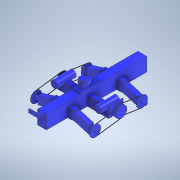
# Autodesk Inventor part: chassis
Saved by Autodesk Inventor 2021 (Build 250183000, 183)
## iProperties
Created: 2020-11-19
Part Number: chassis
Material: Generic
Document SubType Name: Modeling
Designer: Mateusz
Density: 1 g/cm^3
Appearance: Default
Author: Mateusz
Autodesk Inventor part; units mm, degrees
ref_plane "YZ Plane" through (0, 0, 0) normal (1, 0, 0) x (0, 1, 0)
ref_plane "XZ Plane" through (0, 0, 0) normal (0, 1, 0) x (-1, 0, 0)
ref_plane "Work Plane1" through (-479.9998, 3, -645.0001) normal (0, 1, 0) x (1, 0, 0)
sketch "Sketch1" plane through (-479.9998, 3, -645.0001) normal (0, 1, 0) x (1, 0, 0)
  line L0 (-140.0002, -474.9989) -> (-260.0002, -474.9989)
  line L1 (-260.0002, -474.9989) -> (-260.0002, -514.9996)
  line L2 (-260.0002, -514.9996) -> (-380.0002, -544.9996)
  line L3 (-380.0002, -544.9996) -> (-380.0002, -625.0004)
  line L4 (-380.0002, -625.0004) -> (240.0001, -625.0004)
  line L5 (240.0001, -625.0004) -> (240.0001, -545.0003)
  line L6 (240.0001, -545.0003) -> (120.0001, -515.0003)
  line L7 (120.0001, -515.0003) -> (120.0001, -474.9989)
  line L8 (120.0001, -474.9989) -> (0, -474.9989)
  line L9 (0, -474.9989) -> (0.0003, -419.9989)
  line L10 (0.0003, -419.9989) -> (0.0003, -349.9996)
  line L11 (0.0003, -349.9996) -> (-0.0003, -295.0009)
  line L12 (-0.0003, -295.0009) -> (120.0001, -294.9996)
  line L13 (120.0001, -294.9996) -> (120.0001, -255.0003)
  line L14 (120.0001, -255.0003) -> (240, -225)
  line L15 (240, -225) -> (240, -125)
  line L16 (240, -125) -> (120, -95)
  line L17 (120, -95) -> (120, 0)
  line L18 (120, 0) -> (0, 0)
  line L19 (0, 0) -> (0, 70)
  line L20 (0, 70) -> (120, 70)
  line L21 (120, 70) -> (120, 165)
  line L22 (120, 165) -> (240, 195)
  line L23 (240, 195) -> (240, 274.9997)
  line L24 (240, 274.9997) -> (-380.0002, 274.9997)
  line L25 (-380.0002, 274.9997) -> (-380.0002, 194.9997)
  line L26 (-380.0002, 194.9997) -> (-260.0002, 164.9996)
  line L27 (-260.0002, 164.9996) -> (-260.0002, 99.9996)
  line L28 (-260.0002, 99.9996) -> (-260.0002, 70)
  line L29 (-260.0002, 70) -> (-140.0002, 70)
  line L30 (-140.0002, 70) -> (-140.0002, 0)
  line L31 (-140.0002, 0) -> (-260.0002, 0)
  line L32 (-260.0002, 0) -> (-260.0002, -30)
  line L33 (-260.0002, -30) -> (-260.0002, -94.9996)
  line L34 (-260.0002, -94.9996) -> (-380.0002, -124.9996)
  line L35 (-380.0002, -124.9996) -> (-380.0002, -224.9996)
  line L36 (-380.0002, -224.9996) -> (-260.0002, -254.9996)
  line L37 (-260.0002, -254.9996) -> (-260.0002, -294.9996)
  line L38 (-260.0002, -294.9996) -> (-140.0002, -294.9996)
  line L39 (-140.0002, -294.9996) -> (-140.0002, -474.9989)
extrude "Extrusion1" add sketch "Sketch1" along normal blind 3
sketch "Sketch2" plane through (-479.9998, 6, -645.0001) normal (0, 1, 0) x (1, 0, 0)
  line L0 (240, 274.9997) -> (-380.0002, 274.9997) projected
  line L1 (-70.0001, -588.0003) -> (-107.7001, -588.0003)
  line L2 (-107.7001, -588.0003) -> (-32.3001, -588.0003)
  line L3 (-32.3001, -588.0003) -> (-32.3001, 274.9997)
  line L4 (-107.7001, -588.0003) -> (-107.7001, 274.9997)
  line L5 (-32.3001, 274.9997) -> (-107.7001, 274.9997)
  point P0 (479.9998, -645.0001)
  dimension "d4" = 37.7
  dimension "d5" = 75.4
  constraints: 10 end point, 3 point on line, 2 perpendicular, 1 collinear, 1 horizontal
  measures "d4" distance of L1.start L1.end
  measures "d5" distance of L1.end L2.end
extrude "Extrusion2" add sketch "Sketch2" along normal blind 115.4
sketch "Sketch3" plane through (-479.9998, 6, -645.0001) normal (0, 1, 0) x (1, 0, 0)
  line L0 (-140.0002, -404.9993) -> (-107.7001, -404.9993)
  line L1 (-107.7001, -588.0003) -> (-107.7001, 274.9997) projected
  line L2 (-140.0002, -364.9993) -> (0.0003, -364.9993)
  line L3 (0.0003, -404.9993) -> (-107.7001, -404.9993)
  line L4 (0, 15) -> (-140.0002, 15)
  line L5 (-140.0002, 55) -> (0, 55)
  line L6 (-70, -364.9993) -> (28.5, -364.9993)
  line L7 (28.5, -364.9993) -> (-168.5, -364.9993)
  line L8 (-168.5, -364.9993) -> (-168.5, -404.9993)
  line L9 (-168.5, -404.9993) -> (-140.0002, -404.9993)
  line L10 (0.0003, -404.9993) -> (28.5, -404.9993)
  line L11 (28.5, -404.9993) -> (28.5, -364.9993)
  line L12 (0, 55) -> (28.5, 55)
  line L13 (28.5, 55) -> (28.5, 15)
  line L14 (28.5, 15) -> (0, 15)
  line L15 (0, 0) -> (0, 70) projected
  line L16 (-140.0002, 55) -> (-168.5, 55)
  line L17 (-168.5, 55) -> (-168.5, 15)
  line L18 (-168.5, 15) -> (-140.0002, 15)
  point P0 (479.9998, -645.0001)
  dimension "d12" = 40
  dimension "d19" = 98.5
  dimension "d20" = 197
  constraints: 34 end point, 7 point on line, 6 perpendicular, 1 collinear, 1 horizontal, 1 midpoint, 1 parallel
  measures "d12" distance of L4.end L5.start
  measures "d19" distance of L6.start L6.end
  measures "d20" distance of L6.end L7.end
extrude "Extrusion3" add sketch "Sketch3" along normal blind 78.5
sketch "Sketch4" plane through (-479.9998, 6, -645.0001) normal (0, 1, 0) x (1, 0, 0)
  line L0 (0.0003, -404.9993) -> (0.0003, -364.9993) projected
  line L1 (0.0003, -384.9993) -> (0.0003, -349.9993)
  line L2 (0.0003, -349.9993) -> (0.0003, -419.9993)
  line L3 (0, -474.9989) -> (0.0003, -419.9989) projected
  line L4 (0.0003, -419.9993) -> (120.0001, -419.9993)
  line L5 (120.0001, -474.9989) -> (0, -474.9989) projected
  line L6 (120.0001, -419.9993) -> (120.0001, -474.9989)
  line L7 (120.0001, -474.9989) -> (0, -474.9989)
  line L8 (0, -474.9989) -> (0.0003, -419.9993)
  line L9 (0.0003, -419.9989) -> (0.0003, -349.9996) projected
  line L10 (0.0003, -349.9996) -> (-0.0003, -295.0009) projected
  line L11 (0.0003, -349.9996) -> (-0.0003, -295.0009)
  line L12 (-0.0003, -295.0009) -> (120.0001, -294.9996) projected
  line L13 (-0.0003, -295.0009) -> (120.0001, -294.9996)
  line L14 (120.0001, -294.9996) -> (120.0001, -349.9996)
  line L15 (120.0001, -349.9996) -> (0.0003, -349.9996)
  line L16 (-140.0002, -364.9993) -> (-140.0002, -404.9993) projected
  line L17 (-140.0002, -384.9993) -> (-140.0002, -349.9996)
  line L18 (-140.0002, -294.9996) -> (-140.0002, -474.9989) projected
  line L19 (-140.0002, -384.9993) -> (-140.0002, -419.9993)
  line L20 (-140.0002, -294.9996) -> (-140.0002, -474.9989) projected
  arc A0 (-140.0002, -419.9993) -> (-140.0002, -419.9993) centre (-140.0002, 50751.7356) ccw
  line L21 (-140.0002, -419.9993) -> (-140.0002, -474.9989)
  line L22 (-140.0002, -474.9989) -> (-260.0002, -474.9989) projected
  line L23 (-260.0002, -474.9989) -> (-260.0002, -514.9996) projected
  line L24 (-140.0002, -474.9989) -> (-260.0002, -474.9989)
  line L25 (-260.0002, -474.9989) -> (-260.0002, -419.9993)
  line L26 (-260.0002, -419.9993) -> (-140.0002, -419.9993)
  line L27 (-140.0002, -349.9996) -> (-140.0002, -294.9996)
  line L28 (-260.0002, -294.9996) -> (-140.0002, -294.9996) projected
  line L29 (-140.0002, -294.9996) -> (-260.0002, -294.9996)
  line L30 (-260.0002, -294.9996) -> (-260.0002, -349.9996)
  line L31 (-260.0002, -349.9996) -> (-140.0002, -349.9996)
  point P0 (479.9998, -645.0001)
  dimension "d15" = 35
  dimension "d16" = 70
  constraints: 40 end point, 9 point on line, 7 perpendicular, 5 collinear, 2 midpoint, 2 point on circle, 1 centre point, 1 horizontal
  measures "d15" distance of L1.start L1.end
  measures "d16" distance of L1.end L2.end
extrude "Extrusion4" add sketch "Sketch4" against normal up to surface (3 mm away) contours L10 L12 L14 L15 | L31 L30 L28 L18 | L4 L6 L5 L3 | L18 L22 L25 L26
sketch "Sketch5" plane through (-479.9995, 6, -240.0008) normal (0, 0, 1) x (1, 0, 0)
  line L0 (0, 0) -> (28.4997, 0) projected
  line L1 (28.4997, 78.5) -> (-32.3004, 78.5) projected
  line L2 (28.4997, 78.5) -> (28.4997, 68.5)
  line L3 (28.4997, 0) -> (28.4997, 78.5) projected
  line L4 (28.4997, 68.5) -> (150.0967, 31.842)
  line L5 (28.4997, 0) -> (150.0967, -36.658)
  line L6 (150.0967, -36.658) -> (150.0967, 31.842)
  line L7 (28.4997, 68.5) -> (28.4997, 0)
  line L8 (-107.7004, 115.4) -> (-32.3004, 115.4) projected
  line L9 (-70.0004, 115.4) -> (-70.0004, 84.9385)
  line L10 (-140.0008, 0) -> (-168.5005, 0)
  line L11 (-168.5005, 78.5) -> (-107.7004, 78.5)
  line L12 (-168.5005, 78.5) -> (-168.5005, 68.5)
  line L13 (-168.5005, 0) -> (-168.5005, 78.5)
  line L14 (-168.5005, 68.5) -> (-290.0975, 31.842)
  line L15 (-168.5005, 0) -> (-290.0975, -36.658)
  line L16 (-290.0975, -36.658) -> (-290.0975, 31.842)
  line L17 (-168.5005, 68.5) -> (-168.5005, 0)
  point P0 (479.9995, -6)
  dimension "d24" = 10
  constraints: 28 end point, 7 symmetric about line, 2 point on line, 2 vertical, 1 collinear, 1 midpoint, 1 parallel
  measures "d24" distance of L1.start L2.end
extrude "Extrusion5" add sketch "Sketch5" against normal up to surface (40 mm away)
sketch "Sketch6" plane through (-479.9998, 6, -660.0001) normal (0, 0, 1) x (1, 0, 0)
  line L0 (-32.3001, 0) -> (-32.3001, 78.5) projected
  line L1 (0.0003, 0) -> (-32.3001, 0) projected
  line L2 (0.0003, 0) -> (28.5, 0) projected
  line L3 (28.5, 0) -> (150.097, -36.658) projected
  line L4 (150.097, -36.658) -> (150.097, 31.842) projected
  line L5 (150.097, 31.842) -> (28.5, 68.5) projected
  line L6 (28.5, 68.5) -> (28.5, 78.5) projected
  line L7 (-32.3001, 78.5) -> (28.5, 78.5) projected
  line L8 (-290.0972, -36.658) -> (-168.5002, 0) projected
  line L9 (-168.5002, 0) -> (-168.5002, 68.5) projected
  line L10 (-168.5002, 68.5) -> (-290.0972, 31.842) projected
  line L11 (-290.0972, 31.842) -> (-290.0972, -36.658) projected
  point P0 (479.9998, -6)
extrude "Extrusion6" add sketch "Sketch6" against normal up to surface (40 mm away)
sketch "Sketch8" plane through (-479.9998, 121.4, -645.0001) normal (0, 1, 0) x (1, 0, 0)
  line L0 (240, -225) -> (240, -125) projected
  line L1 (240, -175) -> (-32.3001, -174.9996)
  line L2 (-32.3001, 15) -> (-32.3001, -364.9993) projected
  line L3 (-32.3001, -174.9996) -> (-107.7001, -174.9996)
  line L4 (-107.7001, -364.9993) -> (-107.7001, 15) projected
  circle A0 centre (-70.0001, -174.9996) radius 14.9657
  line L5 (-70.0001, -174.9996) -> (-70.0001, -224.9996)
  circle A1 centre (-70.0001, -224.9996) radius 8.3807
  line L6 (-107.7001, 274.9997) -> (-107.7001, -588.0003) projected
  line L7 (-32.3001, -588.0003) -> (-32.3001, 274.9997) projected
  line L8 (-107.7001, -253.6114) -> (-32.3001, -253.6114)
  line L9 (-32.3001, -253.6114) -> (-32.3001, -135.5582)
  line L10 (-32.3001, -135.5582) -> (-107.7001, -135.5582)
  line L11 (-107.7001, -135.5582) -> (-107.7001, -253.6114)
  point P0 (479.9998, -645.0001)
  point P1 (-32.3001, -135.5582)
  point P2 (-107.7001, -135.5582)
  point P3 (-107.7001, -253.6114)
  point P4 (-32.3001, -253.6114)
  dimension "d30" = 50
  constraints: 14 end point, 4 midpoint, 2 centre point, 2 parallel, 2 point on line, 1 coincident, 1 horizontal, 1 perpendicular, 1 vertical
  measures "d30" distance of L5.start L5.end
extrude "Extrusion7" add sketch "Sketch8" along normal blind 13.941 contours L2 L3 A0 L4 L10 | A1 | L2 L8 L4 L3 A0 | A0 L5 L3 | L3 A0 | L5 A0 L3
sketch "Sketch9" plane through (-587.6999, 6, -56.9998) normal (0, 0, 1) x (1, 0, 0)
  line L0 (0, 115.4) -> (75.4, 115.4) projected
  line L1 (37.7, 85.538) -> (47.7, 85.538)
  line L2 (47.7, 85.538) -> (37.7, 85.538)
  line L3 (37.7, 85.538) -> (27.7, 85.538)
  line L4 (27.7, 85.538) -> (27.7, 115.4)
  line L5 (47.7, 85.538) -> (47.7, 115.4)
  line L6 (47.7, 115.4) -> (27.7, 115.4)
  point P0 (587.6999, -6)
  constraints: 12 end point, 3 perpendicular, 3 point on line, 1 collinear, 1 horizontal
extrude "Extrusion8" add sketch "Sketch9" along normal blind 30
sketch "Sketch10" plane through (-587.6999, 6, -26.9998) normal (0, 0, 1) x (1, 0, 0)
  line L0 (47.7, 115.4) -> (27.7, 115.4) projected
  line L1 (47.7, 115.4) -> (53.2, 115.4)
  line L2 (47.7, 115.4) -> (75.4, 115.4) projected
  line L3 (53.2, 115.4) -> (53.2, 85.538)
  line L4 (53.2, 85.538) -> (-40.3, 85.538)
  line L5 (-40.3, 85.538) -> (-40.3, 115.4)
  line L6 (-40.3, 115.4) -> (47.7, 115.4)
  point P0 (587.6999, -6)
  dimension "d39" = 5.5
  dimension "d40" = 93.5
  constraints: 10 end point, 2 perpendicular, 1 collinear, 1 horizontal, 1 point on line
  measures "d39" distance of L0.start L1.end
  measures "d40" distance of L3.end L4.end
extrude "Extrusion9" add sketch "Sketch10" along normal blind 7
sketch "Sketch11" plane through (-479.9998, 6, -645.0001) normal (0, 1, 0) x (1, 0, 0)
  line L0 (-107.7001, -404.9993) -> (-140.0002, -404.9993) projected
  line L1 (-140.0002, -404.9993) -> (-140.0002, -419.9993) projected
  line L2 (-140.0002, -419.9993) -> (-260.0002, -419.9993) projected
  line L3 (-260.0002, -419.9993) -> (-260.0002, -514.9996) projected
  line L4 (-260.0002, -514.9996) -> (-380.0002, -544.9996) projected
  line L5 (-380.0002, -544.9996) -> (-380.0002, -625.0004) projected
  line L6 (-380.0002, -625.0004) -> (240.0001, -625.0004) projected
  line L7 (240.0001, -625.0004) -> (240.0001, -545.0003) projected
  line L8 (240.0001, -545.0003) -> (120.0001, -515.0003) projected
  line L9 (120.0001, -515.0003) -> (120.0001, -419.9993) projected
  line L10 (120.0001, -419.9993) -> (0.0003, -419.9993) projected
  line L11 (0.0003, -419.9993) -> (0.0003, -419.9989) projected
  line L12 (0.0003, -419.9989) -> (0.0003, -404.9993) projected
  line L13 (0.0003, -404.9993) -> (-32.3001, -404.9993) projected
  line L14 (-32.3001, -404.9993) -> (-32.3001, -588.0003) projected
  line L15 (-32.3001, -588.0003) -> (-107.7001, -588.0003) projected
  line L16 (-107.7001, -588.0003) -> (-107.7001, -404.9993) projected
  line L17 (-107.7001, 15) -> (-140.0002, 15) projected
  line L18 (-140.0002, 15) -> (-140.0002, 0) projected
  line L19 (-140.0002, 0) -> (-260.0002, 0) projected
  line L20 (-260.0002, 0) -> (-260.0002, -94.9996) projected
  line L21 (-260.0002, -94.9996) -> (-380.0002, -124.9996) projected
  line L22 (-380.0002, -124.9996) -> (-380.0002, -224.9996) projected
  line L23 (-380.0002, -224.9996) -> (-260.0002, -254.9996) projected
  line L24 (-260.0002, -254.9996) -> (-260.0002, -349.9996) projected
  line L25 (-260.0002, -349.9996) -> (-140.0002, -349.9996) projected
  line L26 (-140.0002, -349.9996) -> (-140.0002, -364.9993) projected
  line L27 (-140.0002, -364.9993) -> (-107.7001, -364.9993) projected
  line L28 (-107.7001, -364.9993) -> (-107.7001, 15) projected
  line L29 (-140.0002, 55) -> (-107.7001, 55) projected
  line L30 (-107.7001, 55) -> (-107.7001, 274.9997) projected
  line L31 (-107.7001, 274.9997) -> (-380.0002, 274.9997) projected
  line L32 (-380.0002, 274.9997) -> (-380.0002, 194.9997) projected
  line L33 (-380.0002, 194.9997) -> (-260.0002, 164.9996) projected
  line L34 (-260.0002, 164.9996) -> (-260.0002, 70) projected
  line L35 (-260.0002, 70) -> (-140.0002, 70) projected
  line L36 (-140.0002, 70) -> (-140.0002, 55) projected
  line L37 (-32.3001, 55) -> (0, 55) projected
  line L38 (0, 55) -> (0, 70) projected
  line L39 (0, 70) -> (120, 70) projected
  line L40 (120, 70) -> (120, 165) projected
  line L41 (120, 165) -> (240, 195) projected
  line L42 (240, 195) -> (240, 274.9997) projected
  line L43 (240, 274.9997) -> (-32.3001, 274.9997) projected
  line L44 (-32.3001, 274.9997) -> (-32.3001, 55) projected
  line L45 (0, 15) -> (-32.3001, 15) projected
  line L46 (-32.3001, 15) -> (-32.3001, -364.9993) projected
  line L47 (-32.3001, -364.9993) -> (0.0003, -364.9993) projected
  line L48 (0.0003, -364.9993) -> (0.0003, -349.9996) projected
  line L49 (0.0003, -349.9996) -> (120.0001, -349.9996) projected
  line L50 (120.0001, -349.9996) -> (120.0001, -255.0003) projected
  line L51 (120.0001, -255.0003) -> (240, -225) projected
  line L52 (240, -225) -> (240, -125) projected
  line L53 (240, -125) -> (120, -95) projected
  line L54 (120, -95) -> (120, 0) projected
  line L55 (120, 0) -> (0, 0) projected
  line L56 (0, 0) -> (0, 15) projected
  point P0 (479.9998, -645.0001)
extrude "Extrusion10" cut sketch "Sketch11" against normal up to surface (3 mm away)
sketch "Sketch13" plane through (-479.9998, 121.4, -645.0001) normal (0, 1, 0) x (1, 0, 0)
  line L0 (-32.3001, -253.6114) -> (-107.7001, -253.6114) projected
  line L1 (-32.3001, -253.6114) -> (-32.3001, -293.6114)
  line L2 (-32.3001, -588.0003) -> (-32.3001, -253.6114) projected
  line L3 (-32.3001, -293.6114) -> (-107.7001, -293.6114)
  line L4 (-107.7001, -364.9993) -> (-107.7001, 15) projected
  line L5 (-107.7001, -253.6114) -> (-107.7001, -293.6114)
  point P0 (479.9998, -645.0001)
  dimension "d45" = 40
  constraints: 6 end point, 3 point on line, 1 collinear, 1 perpendicular
  measures "d45" distance of L0.start L1.end
extrude "Extrusion11" add sketch "Sketch13" along normal up to surface (13.941 mm away)
sketch "Sketch14" plane through (-479.9998, 135.341, -645.0001) normal (0, 1, 0) x (1, 0, 0)
  line L0 (-32.3001, -293.6114) -> (-107.7001, -293.6114) projected
  circle A0 centre (-70.0001, -237.6499) radius 30.3987
  circle A1 centre (-70.0001, -178.6114) radius 12.4726
  line L1 (-98.9637, -228.4198) -> (-81.8838, -174.8243)
  line L2 (-41.0365, -228.4198) -> (-58.1164, -174.8243)
  point P0 (479.9998, -645.0001)
  constraints: 4 end point, 4 point on circle, 4 tangent, 2 centre point, 1 other
extrude "Extrusion12" add sketch "Sketch14" along normal blind 40
sketch "Sketch15" plane through (-479.9998, 175.341, -645.0001) normal (0, 1, 0) x (1, 0, 0)
  arc A0 (-98.9637, -228.4198) -> (-41.0365, -228.4198) centre (-70.0001, -237.6499) ccw projected
  circle A1 centre (-70.0001, -237.6499) radius 27.858
  point P0 (479.9998, -645.0001)
  constraints: 1 centre point, 1 coincident
extrude "Extrusion13" add sketch "Sketch15" along normal blind 20
sketch "Sketch16" plane through (-587.6999, 3, -56.9998) normal (-1, 0, 0) x (0, 0, 1)
  line L0 (-223.0011, 3) -> (-223.0011, 81.5) projected
  line L1 (-223.0011, 81.5) -> (-353.0011, 81.5)
  line L2 (-353.0011, 81.5) -> (-353.0011, 0)
  line L3 (-603.0003, 0) -> (-223.0011, 0) projected
  line L4 (-353.0011, 81.5) -> (-393.0011, 81.5)
  line L5 (-393.0011, 81.5) -> (-393.0011, 0)
  line L6 (-353.0011, 0) -> (-393.0011, 0)
  point P0 (56.9998, -3)
  dimension "d55" = 130
  dimension "d56" = 40
  constraints: 10 end point, 3 perpendicular, 3 point on line, 1 horizontal
  measures "d55" distance of L0.end L1.end
  measures "d56" distance of L1.end L4.end
extrude "Extrusion14" add sketch "Sketch16" along normal up to surface (182.3971 mm away)
sketch "Sketch17" plane through (-770.097, 3, -450.0008) normal (-1, 0, 0) x (0, 0, 1)
  line L0 (40, 0) -> (0, 0) projected
  line L1 (40, 0) -> (40, 90)
  line L2 (40, 90) -> (-85, 90)
  line L3 (-85, 90) -> (-85, 0)
  line L4 (-209.9993, 0) -> (170, 0) projected
  line L5 (40, 0) -> (-85, 0)
  point P0 (450.0008, -3)
  dimension "d59" = 90
  dimension "d60" = 125
  constraints: 8 end point, 3 perpendicular, 1 point on line, 1 vertical
  measures "d59" distance of L0.start L1.end
  measures "d60" distance of L1.end L2.end
extrude "Extrusion15" add sketch "Sketch17" against normal blind 3
sketch "Sketch18" plane through (-587.6999, 3, -410.0008) normal (0, 0, 1) x (1, 0, 0)
  line L0 (-179.3971, 0) -> (-179.3971, 81.5) projected
  line L1 (0, 81.5) -> (-179.3971, 81.5) projected
  line L2 (-179.3971, 81.5) -> (-149.3971, 81.5)
  circle A0 centre (-149.3971, 81.5) radius 30
  point P0 (587.6999, -3)
  dimension "d64" = 30
  constraints: 2 end point, 1 coincident, 1 horizontal alignment, 1 point on line, 2 other
  measures "d64" distance of L0.end L2.end
extrude "Extrusion16" add sketch "Sketch18" along normal blind 60
extrude "Extrusion17" add sketch "Sketch18" against normal blind 100
sketch "Sketch19" plane through (-512.2999, 3, -919.9998) normal (1, 0, 0) x (0, 0, -1)
  line L0 (-469.9989, 81.5) -> (-509.9989, 81.5) projected
  line L1 (-469.9989, 0) -> (-469.9989, 81.5) projected
  line L2 (-509.9989, 81.5) -> (-509.9989, 0) projected
  line L3 (-469.9989, 0) -> (-259.9997, 0) projected
  line L4 (-219.9997, 0) -> (-259.9997, 0) projected
  line L5 (-219.9997, 0) -> (0, 0) projected
  line L6 (0, 0) -> (-219.9997, 0) projected
  line L7 (-259.9997, 0) -> (-219.9997, 0) projected
  line L8 (-259.9997, 0) -> (-639.9989, 0) projected
  line L9 (-679.9989, 0) -> (-639.9989, 0) projected
  line L10 (-679.9989, 0) -> (-863, 0) projected
  line L11 (-863, 0) -> (-679.9989, 0) projected
  line L12 (-639.9989, 0) -> (-679.9989, 0) projected
  line L13 (-639.9989, 0) -> (-509.9989, 0) projected
  line L14 (-509.9989, 0) -> (-384.9989, 0) projected
  line L15 (-469.9989, 0) -> (-384.9989, 0) projected
  point P0 (-919.9998, -3)
  point P1 (-509.9989, 0)
extrude "Extrusion18" add sketch "Sketch19" along normal up to surface (182.3971 mm away)
sketch "Sketch20" plane through (-329.9028, 3, -410.0008) normal (1, 0, 0) x (0, 0, -1)
  line L0 (40, 0) -> (40, 81.5) projected
  line L1 (0, 0) -> (125, 0) projected
  line L2 (0, 0) -> (0, 90) projected
  line L3 (0, 90) -> (125, 90) projected
  line L4 (125, 90) -> (125, 0) projected
  point P0 (-410.0008, -3)
extrude "Extrusion19" add sketch "Sketch20" against normal blind 3
sketch "Sketch21" plane through (-512.2999, 3, -450.0008) normal (0, 0, -1) x (-1, 0, 0)
  line L0 (0, 81.5) -> (-179.3971, 81.5) projected
  line L1 (-179.3971, 81.5) -> (-149.3971, 81.5)
  circle A0 centre (-149.3971, 81.5) radius 30
  point P0 (-512.2999, -3)
  dimension "d73" = 30
  constraints: 2 end point, 1 coincident, 1 horizontal alignment, 1 point on line, 2 other
  measures "d73" distance of L0.end L1.end
extrude "Extrusion20" add sketch "Sketch21" along normal up to surface (60 mm away)
extrude "Extrusion21" add sketch "Sketch21" against normal up to surface (100 mm away)
sketch "Sketch22" plane through (-329.9028, -30.658, -240.0008) normal (1, 0, 0) x (0, 0, -1)
  line L0 (0, 68.5) -> (40, 68.5) projected
  line L1 (20, 68.5) -> (20, 0)
  line L2 (0, 0) -> (40, 0) projected
  line L3 (40, 0) -> (40, 68.5) projected
  line L4 (40, 34.25) -> (0, 34.25)
  line L5 (0, 0) -> (0, 68.5) projected
  circle A0 centre (20, 34.25) radius 15
  point P0 (-240.0008, 30.658)
  dimension "d78" = 30
  constraints: 5 midpoint, 4 end point, 1 centre point
  measures "d78" diameter of A0
extrude "Extrusion22" add sketch "Sketch22" along normal blind 50.5 contours A0 L4 L1 | L1 L4 A0 | L4 L1 A0 | L4 A0 L1
sketch "Sketch23" plane through (-329.9028, -30.658, -660.0001) normal (1, 0, 0) x (0, 0, -1)
  line L0 (0, 68.5) -> (40, 68.5) projected
  line L1 (20, 68.5) -> (20, 0)
  line L2 (0, 0) -> (40, 0) projected
  line L3 (40, 0) -> (40, 68.5) projected
  line L4 (40, 34.25) -> (0, 34.25)
  line L5 (0, 0) -> (0, 68.5) projected
  circle A0 centre (20, 34.25) radius 15
  point P0 (-660.0001, 30.658)
  dimension "d81" = 30
  constraints: 5 midpoint, 4 end point, 1 centre point
  measures "d81" diameter of A0
extrude "Extrusion23" add sketch "Sketch23" along normal up to surface (50.5 mm away) contours A0 L4 L1 | L1 L4 A0 | L4 L1 A0 | L4 A0 L1
sketch "Sketch24" plane through (-770.097, -30.658, -240.0008) normal (-1, 0, 0) x (0, 0, 1)
  line L0 (0, 0) -> (-40, 0) projected
  line L1 (-20, 0) -> (-20, 68.5)
  line L2 (0, 68.5) -> (-40, 68.5) projected
  line L3 (0, 68.5) -> (0, 0) projected
  line L4 (0, 34.25) -> (-40, 34.25)
  line L5 (-40, 68.5) -> (-40, 0) projected
  line L6 (-419.9993, 68.5) -> (-459.9993, 68.5) projected
  line L7 (-439.9993, 68.5) -> (-439.9993, 0)
  line L8 (-419.9993, 0) -> (-459.9993, 0) projected
  line L9 (-419.9993, 68.5) -> (-419.9993, 0) projected
  line L10 (-419.9993, 34.25) -> (-459.9993, 34.25)
  line L11 (-459.9993, 68.5) -> (-459.9993, 0) projected
  circle A0 centre (-439.9993, 34.25) radius 15
  circle A1 centre (-20, 34.25) radius 15
  point P0 (240.0008, 30.658)
  dimension "d84" = 30
  dimension "d85" = 30
  constraints: 10 midpoint, 8 end point, 2 centre point
  measures "d84" diameter of A0
  measures "d85" diameter of A1
extrude "Extrusion24" add sketch "Sketch24" along normal blind 50.5 contours A1 L4 L1 | L1 L4 A1 | L4 L1 A1 | L4 A1 L1 | A0 L10 L7 | L7 L10 A0 | A0 L7 L10 | L7 A0 L10
ref_plane "Work Plane2" through (-294.4028, 3.592, -260.0008) normal (1, 0, 0) x (0, 0, -1)
ref_plane "Work Plane3" through (-805.597, 3.592, -260.0008) normal (-1, 0, 0) x (0, 0, 1)
sketch "Sketch25" plane through (-294.4028, 3.592, -260.0008) normal (1, 0, 0) x (0, 0, -1)
  circle A0 centre (0, 0) radius 15 projected
  circle A1 centre (0, 0) radius 47.5
  circle A2 centre (419.9993, 0) radius 15 projected
  circle A3 centre (419.9993, 0) radius 47.5
  point P0 (-260.0008, -3.592)
  dimension "d90" = 95
  dimension "d93" = 95
  constraints: 2 centre point, 2 coincident
  measures "d90" diameter of A1
  measures "d93" diameter of A3
extrude "Extrusion25" add sketch "Sketch25" against normal blind 3 contours A1
sketch "Sketch26" plane through (-805.597, 3.592, -260.0008) normal (-1, 0, 0) x (0, 0, 1)
  circle A0 centre (0, 0) radius 15 projected
  circle A1 centre (0, 0) radius 47.5
  point P0 (260.0008, -3.592)
  dimension "d94" = 95
  constraints: 1 centre point, 1 coincident
  measures "d94" diameter of A1
extrude "Extrusion26" add sketch "Sketch26" against normal blind 3
ref_plane "Work Plane4" through (-314.4028, 3.592, -680.0001) normal (1, 0, 0) x (0, 0, -1)
sketch "Sketch27" plane through (-314.4028, 3.592, -680.0001) normal (1, 0, 0) x (0, 0, -1)
  circle A0 centre (0, 0) radius 15 projected
  circle A1 centre (0, 0) radius 47.5
  point P0 (-680.0001, -3.592)
  dimension "d98" = 95
  constraints: 1 centre point, 1 coincident
  measures "d98" diameter of A1
extrude "Extrusion27" add sketch "Sketch27" along normal blind 3
ref_plane "Work Plane5" through (-785.597, 3.592, -680.0001) normal (-1, 0, 0) x (0, 0, 1)
sketch "Sketch28" plane through (-785.597, 3.592, -680.0001) normal (-1, 0, 0) x (0, 0, 1)
  circle A0 centre (0, 0) radius 15 projected
  circle A1 centre (0, 0) radius 47.5
  point P0 (680.0001, -3.592)
  dimension "d102" = 95
  constraints: 1 centre point, 1 coincident
  measures "d102" diameter of A1
extrude "Extrusion28" add sketch "Sketch28" along normal blind 3
sketch "Sketch29" plane through (-770.097, 3, -535.0008) normal (-1, 0, 0) x (0, 0, 1)
  line L0 (0, 90) -> (0, 0) projected
  circle A0 centre (50, 30) radius 12.5
  point P0 (535.0008, -3)
  dimension "d108" = 25
  constraints: 1 centre point
  measures "d108" diameter of A0
extrude "Extrusion29" add sketch "Sketch29" along normal up to surface (35.5 mm away)
ref_plane "Work Plane6" through (-788.597, 33, -485.0008) normal (-1, 0, 0) x (0, 0, 1)
sketch "Sketch30" plane through (-788.597, 33, -485.0008) normal (-1, 0, 0) x (0, 0, 1)
  circle A0 centre (0, 0) radius 12.5 projected
  circle A1 centre (0, 0) radius 47.5
  point P0 (485.0008, -33)
  dimension "d112" = 95
  constraints: 1 centre point, 1 coincident
  measures "d112" diameter of A1
extrude "Extrusion30" add sketch "Sketch30" against normal up to surface (3 mm away)
sketch "Sketch31" plane through (-805.597, 33, -485.0008) normal (-1, 0, 0) x (0, 0, 1)
  circle A0 centre (0, 0) radius 12.5 projected
  circle A1 centre (0, 0) radius 47.5
  point P0 (485.0008, -33)
  constraints: 1 centre point, 1 coincident
extrude "Extrusion31" add sketch "Sketch31" against normal up to surface (3 mm away)
sketch "Sketch32" plane through (-329.9028, 3, -535.0008) normal (1, 0, 0) x (0, 0, -1)
  circle A0 centre (-50, 30) radius 12.5 projected
  point P0 (-535.0008, -3)
extrude "Extrusion32" add sketch "Sketch32" along normal blind 35.5
ref_plane "Work Plane7" through (-311.4028, 33, -485.0008) normal (1, 0, 0) x (0, 0, -1)
sketch "Sketch33" plane through (-311.4028, 33, -485.0008) normal (1, 0, 0) x (0, 0, -1)
  circle A0 centre (0, 0) radius 12.5 projected
  circle A1 centre (0, 0) radius 47.5
  point P0 (-485.0008, -33)
  dimension "d120" = 95
  constraints: 1 centre point, 1 coincident
  measures "d120" diameter of A1
extrude "Extrusion33" add sketch "Sketch33" against normal up to surface (3 mm away)
sketch "Sketch34" plane through (-294.4028, 33, -485.0008) normal (1, 0, 0) x (0, 0, -1)
  circle A0 centre (0, 0) radius 12.5 projected
  circle A1 centre (0, 0) radius 47.5
  point P0 (-485.0008, -33)
  dimension "d123" = 95
  constraints: 1 centre point, 1 coincident
  measures "d123" diameter of A1
extrude "Extrusion34" add sketch "Sketch34" against normal up to surface (3 mm away)
sketch "Sketch35" plane through (-294.4028, 3.592, -260.0008) normal (1, 0, 0) x (0, 0, -1)
  circle A0 centre (0, 0) radius 47.5 projected
  circle A1 centre (0, 0) radius 15 projected
  circle A2 centre (225, 29.408) radius 47.5 projected
  circle A3 centre (0, 0) radius 47.5 projected
  line L0 (-6.156, 47.0994) -> (218.844, 76.5074)
  circle A4 centre (225, 29.408) radius 47.5 projected
  line L1 (6.156, -47.0994) -> (231.156, -17.6914)
  line L2 (218.844, 76.5074) -> (219.168, 74.0285)
  line L3 (219.168, 74.0285) -> (-5.832, 44.6205)
  line L4 (-5.832, 44.6205) -> (-6.156, 47.0994)
  line L5 (231.156, -17.6914) -> (230.832, -15.2125)
  line L6 (230.832, -15.2125) -> (5.832, -44.6205)
  line L7 (5.832, -44.6205) -> (6.156, -47.0994)
  point P0 (-260.0008, -3.592)
  point P1 (9.2467, 46.5913)
  point P2 (204.0893, 72.0577)
  point P3 (218.844, 76.5074)
  point P4 (-6.156, 47.0994)
  dimension "d126" = 2.5
  dimension "d127" = 2.5
  constraints: 16 end point, 4 perpendicular, 12 other
  measures "d126" distance of L0.end L2.end
  measures "d127" distance of L1.end L5.end
extrude "Extrusion35" add sketch "Sketch35" against normal up to surface (3 mm away) contours L0 A2 L3 A0 | L7 L6 A0 | A0 L6 A2 L1 | A2 L6 L5
sketch "Sketch36" plane through (-311.4028, 3.592, -680.0001) normal (1, 0, 0) x (0, 0, -1)
  arc A0 (-188.8433, -17.6914) -> (-201.1553, 76.5074) centre (-194.9993, 29.408) ccw projected
  line L0 (-201.1553, 76.5074) -> (-426.1553, 47.0994) projected
  arc A1 (-426.1553, 47.0994) -> (-413.8433, -47.0994) centre (-419.9993, 0) ccw projected
  line L1 (-413.8433, -47.0994) -> (-188.8433, -17.6914) projected
  circle A2 centre (-419.9993, 0) radius 15 projected
  line L2 (-204.2459, -17.1833) -> (-399.0886, -42.6497) projected
  arc A3 (-399.0886, -42.6497) -> (-410.7526, 46.5913) centre (-419.9993, 0) ccw projected
  line L3 (-410.7526, 46.5913) -> (-215.9099, 72.0577) projected
  arc A4 (-215.9099, 72.0577) -> (-204.2459, -17.1833) centre (-194.9993, 29.408) ccw projected
  circle A5 centre (0, 0) radius 47.5 projected
  circle A6 centre (0, 0) radius 15 projected
  circle A7 centre (0, 0) radius 47.5 projected
  line L4 (0, 47.5) -> (-187.7846, 76.3569)
  arc A8 (-188.8433, -17.6914) -> (-201.1553, 76.5074) centre (-194.9993, 29.408) ccw projected
  line L5 (0, -47.5) -> (-191.6179, -18.054)
  line L6 (-188.8433, -17.6914) -> (-413.8433, -47.0994) projected
  line L7 (0, 47.5) -> (-0.3797, 45.029)
  line L8 (-0.3797, 45.029) -> (-188.1644, 73.8859)
  line L9 (-187.7846, 76.3569) -> (-188.1644, 73.8859)
  line L10 (0, -47.5) -> (0.3797, -45.029)
  line L11 (0.3797, -45.029) -> (-191.2391, -15.5829)
  line L12 (-191.6179, -18.054) -> (-191.2382, -15.5831)
  line L13 (-191.2382, -15.5831) -> (-183.7325, -16.7364)
  point P0 (-680.0001, -3.592)
  point P1 (-23.3064, -41.3892)
  point P2 (-183.7325, -16.7364)
  point P3 (-191.6179, -18.054)
  point P4 (-14.2619, -45.3084)
  dimension "d130" = 2.5
  dimension "d131" = 2.5
  dimension "d132" = 2.5
  constraints: 18 end point, 4 parallel, 3 point on line, 2 perpendicular, 2 point on circle, 1 tangent, 1 vertical alignment, 3 other
  measures "d130" distance of L4.start L7.end
  measures "d131" distance of L5.start L10.end
  measures "d132" distance of L5.end L12.end
extrude "Extrusion36" add sketch "Sketch36" against normal up to surface (3 mm away) contours A0 L11 A5 L5 L1 | L8 L9 A0 | A0 L4 A5 L8 | A5 L7 L8
sketch "Sketch37" plane through (-788.597, 3.592, -680.0001) normal (-1, 0, 0) x (0, 0, 1)
  arc A0 (188.8433, -17.6914) -> (187.7846, 76.3569) centre (194.9993, 29.408) ccw projected
  line L0 (187.7846, 76.3569) -> (0, 47.5) projected
  arc A1 (0, 47.5) -> (14.2619, -45.3084) centre (0, 0) ccw projected
  line L1 (14.2619, -45.3084) -> (191.6179, -18.054) projected
  line L2 (191.6179, -18.054) -> (188.8433, -17.6914) projected
  circle A2 centre (0, 0) radius 15 projected
  line L3 (183.7325, -16.7364) -> (23.3064, -41.3892) projected
  arc A3 (23.3064, -41.3892) -> (9.8039, 46.4772) centre (0, 0) ccw projected
  line L4 (9.8039, 46.4772) -> (173.1339, 71.5762) projected
  arc A4 (173.1339, 71.5762) -> (183.7325, -16.7364) centre (194.9993, 29.408) ccw projected
  circle A5 centre (194.9993, 29.408) radius 12.5 projected
  point P0 (680.0001, -3.592)
extrude "Extrusion37" add sketch "Sketch37" against normal up to surface (3 mm away)
sketch "Sketch38" plane through (-805.597, 3.592, -260.0008) normal (-1, 0, 0) x (0, 0, 1)
  arc A0 (-215.7533, -17.1833) -> (-204.0893, 72.0577) centre (-225, 29.408) ccw projected
  line L0 (-204.0893, 72.0577) -> (-9.2467, 46.5913) projected
  arc A1 (-9.2467, 46.5913) -> (-20.9107, -42.6497) centre (0, 0) ccw projected
  line L1 (-20.9107, -42.6497) -> (-215.7533, -17.1833) projected
  circle A2 centre (0, 0) radius 15 projected
  line L2 (-231.156, -17.6914) -> (-6.156, -47.0994) projected
  arc A3 (-6.156, -47.0994) -> (6.156, 47.0994) centre (0, 0) ccw projected
  line L3 (6.156, 47.0994) -> (-218.844, 76.5074) projected
  arc A4 (-218.844, 76.5074) -> (-231.156, -17.6914) centre (-225, 29.408) ccw projected
  circle A5 centre (-225, 29.408) radius 12.5 projected
  point P0 (260.0008, -3.592)
extrude "Extrusion38" add sketch "Sketch38" against normal up to surface (3 mm away)
equation "\"d82\" = d81"
body "Solid2"
